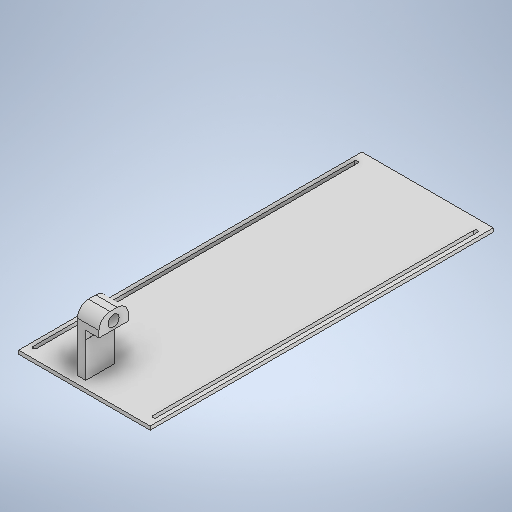
# Autodesk Inventor part: Part1
Saved by Autodesk Inventor 2025.2 (Build 292293000, 293)
## iProperties
Created: 2026-09-08
Part Number: Part1
Material: Generic
Document SubType Name: Sheet Metal
Designer: dguar
Density: 1 g/cm^3
Sheet Metal Rule: Default_mm
Appearance: Default
Author: dguar
Autodesk Inventor part; units mm, degrees
ref_plane "YZ Plane" through (0, 0, 0) normal (1, 0, 0) x (0, 1, 0)
ref_plane "XZ Plane" through (0, 0, 0) normal (0, 1, 0) x (-1, 0, 0)
ref_plane "XY Plane" through (0, 0, 0) normal (0, 0, 1) x (1, 0, 0)
sketch "Sketch1" plane through (0, 0, 0) normal (0, 1, 0) x (-1, 0, 0)
  line L0 (80, 0) -> (80, -250)
  line L1 (80, -250) -> (-80, -250)
  line L2 (-80, -250) -> (-80, 250)
  line L3 (-80, 250) -> (80, 250)
  line L4 (80, 250) -> (80, 0)
  point P0 (0, 0)
  constraints: 10 end point, 2 perpendicular, 1 point on line, 1 vertical
extrude "Extrusion1" add sketch "Sketch1" along normal blind 5
sketch "Sketch2" plane through (0, 5, 0) normal (0, 1, 0) x (1, 0, 0)
  line L0 (0, 0) -> (0, -200)
  line L1 (0, -200) -> (10, -200)
  line L2 (10, -200) -> (-10, -200)
  line L3 (-10, -200) -> (-10, -240)
  line L4 (-10, -240) -> (10, -240)
  line L5 (10, -240) -> (10, -200)
  dimension "d7" = 200
  dimension "d8" = 10
  dimension "d9" = 20
  dimension "d10" = 40
  dimension "d11" = 20
  constraints: 12 end point, 2 perpendicular, 1 horizontal, 1 point on line, 1 vertical
  measures "d7" distance of L0.start L0.end
  measures "d8" distance of L0.end L1.end
  measures "d9" distance of L1.end L2.end
  measures "d10" distance of L2.end L3.end
  measures "d11" distance of L3.end L4.end
extrude "Extrusion2" add sketch "Sketch2" along normal blind 100
sketch "Sketch3" plane through (10, 5, 240) normal (1, 0, 0) x (0, 0, -1)
  line L0 (40, 100) -> (0, 100) projected
  circle A0 centre (20, 70) radius 7.5
  point P0 (240, -5)
  dimension "d15" = 15
  constraints: 1 centre point
  measures "d15" diameter of A0
extrude "Extrusion3" cut sketch "Sketch3" against normal blind 100
sketch "Sketch4" plane through (80, 0, 250) normal (1, 0, 0) x (0, 0, -1)
  line L0 (0, 0) -> (0, 5) projected
  line L1 (0, 0) -> (500, 0) projected
  line L2 (0, 5) -> (500, 5)
  line L3 (500, 5) -> (500, 0)
  line L4 (500, 0) -> (0, 0)
  line L5 (0, 0) -> (0, 5)
  point P0 (250, 0)
  constraints: 8 end point, 2 parallel, 1 horizontal, 1 perpendicular
extrude "Extrusion4" add sketch "Sketch4" along normal blind 10
sketch "Sketch5" plane through (-80, 0, -250) normal (-1, 0, 0) x (0, 0, 1)
  line L0 (0, 5) -> (500, 5) projected
  line L1 (500, 0) -> (500, 5) projected
  line L2 (0, 5) -> (500, 5)
  line L3 (500, 5) -> (500, 0)
  line L4 (500, 0) -> (0, 0)
  line L5 (0, 0) -> (0, 5)
  point P0 (250, 0)
  constraints: 8 end point, 2 parallel, 1 horizontal, 1 perpendicular
extrude "Extrusion5" add sketch "Sketch5" along normal blind 10
sketch "Sketch6" plane through (90, 0, -250) normal (0, 0, -1) x (-1, 0, 0)
  line L0 (0, 5) -> (180, 5) projected
  line L1 (180, 0) -> (0, 0) projected
  line L2 (0, 5) -> (180, 5)
  line L3 (180, 5) -> (180, 0)
  line L4 (180, 0) -> (0, 0)
  line L5 (0, 0) -> (0, 5)
  point P0 (90, 0)
  constraints: 8 end point, 2 parallel, 1 horizontal, 1 perpendicular
extrude "Extrusion6" cut sketch "Sketch6" against normal blind 30
sketch "Sketch7" plane through (0, 5, 0) normal (0, 1, 0) x (1, 0, 0)
  line L0 (-90, -250) -> (90, -250) projected
  arc A0 (79.52, -235.7841) -> (84.52, -235.7841) centre (82.02, -235.7841) ccw
  arc A1 (84.52, 203.719) -> (79.52, 203.719) centre (82.02, 203.719) ccw
  line L1 (79.52, 203.719) -> (79.52, -235.7841)
  line L2 (84.52, -235.7841) -> (84.52, 203.719)
  line L3 (-90, -250) -> (-90, 220) projected
  line L4 (90, 220) -> (-90, 220) projected
  arc A2 (-79.52, 203.719) -> (-84.52, 203.719) centre (-82.02, 203.719) ccw
  arc A3 (-84.52, -235.7841) -> (-79.52, -235.7841) centre (-82.02, -235.7841) ccw
  line L5 (-84.52, -235.7841) -> (-84.52, 203.719)
  line L6 (-79.52, 203.719) -> (-79.52, -235.7841)
  point P0 (0, 0)
  dimension "d25" = 5
  dimension "d26" = 5
  dimension "d28" = 5
  dimension "d29" = 5
  constraints: 8 end point, 8 point on circle, 4 centre point, 4 tangent
  measures "d25" diameter of A0
  measures "d26" diameter of A1
  measures "d28" diameter of A2
  measures "d29" diameter of A3
extrude "Extrusion7" cut sketch "Sketch7" against normal blind 30
sketch "Sketch8" plane through (10, 5, 240) normal (1, 0, 0) x (0, 0, -1)
  point P0 (240, -5)
sketch "Sketch9" plane through (0, 105, 0) normal (0, 1, 0) x (1, 0, 0)
  line L0 (10, -240) -> (-10, -240) projected
  line L1 (-10, -200) -> (10, -200) projected
  line L2 (-10, -240) -> (10, -240)
  line L3 (10, -240) -> (10, -200)
  line L4 (10, -200) -> (-10, -200)
  line L5 (-10, -200) -> (-10, -240)
  point P0 (0, 0)
  constraints: 8 end point, 2 parallel, 1 horizontal, 1 perpendicular
extrude "Extrusion8" cut sketch "Sketch9" against normal blind 16.75
sketch "Sketch10" plane through (-10, 5, 200) normal (-1, 0, 0) x (0, 0, 1)
  line L0 (0, 0) -> (0, 83.25) projected
  line L1 (40, 0) -> (40, 83.25) projected
  line L2 (0, 83.25) -> (40, 83.25)
  line L3 (40, 83.25) -> (40, 0)
  line L4 (40, 0) -> (0, 0)
  line L5 (0, 0) -> (0, 83.25)
  circle A0 centre (20, 70) radius 7.5 projected
  circle A1 centre (20, 70) radius 7.5
  point P0 (-200, -5)
  constraints: 8 end point, 2 parallel, 1 centre point, 1 coincident, 1 horizontal, 1 perpendicular
extrude "Extrusion9" add sketch "Sketch10" along normal blind 9.5
sketch "Sketch11" plane through (10, 5, 200) normal (0, 0, -1) x (-1, 0, 0)
  line L0 (0, 0) -> (0, 83.25) projected
  line L1 (0, 0) -> (18.187, 0)
  line L2 (18.187, 0) -> (18.187, 48.2097)
  line L3 (18.187, 48.2097) -> (0, 48.2097)
  line L4 (0, 48.2097) -> (0, 0)
  point P0 (10, -5)
  constraints: 8 end point, 2 parallel, 1 horizontal, 1 perpendicular
extrude "Extrusion10" cut sketch "Sketch11" against normal blind 66.75
sketch "Sketch12" plane through (10, 88.25, 240) normal (1, 0, 0) x (0, 0, -1)
  line L0 (0, -83.25) -> (0, 0) projected
  line L1 (40, 0) -> (40, -83.25) projected
  line L2 (0, -35.059) -> (40, -35.059)
  line L3 (40, -35.059) -> (40, -23.8514)
  line L4 (40, -23.8514) -> (0, -23.8514)
  line L5 (0, -23.8514) -> (0, -35.059)
  point P0 (240, -88.25)
  constraints: 8 end point, 2 parallel, 2 point on line, 1 horizontal, 1 perpendicular
extrude "Extrusion11" cut sketch "Sketch12" against normal blind 18.25
fillet "Fillet1" radius 15 2 edges at (-4.75, 88.25, 240) (-4.75, 88.25, 200)
equation "\"BendRadius\" = Thickness"
equation "\"BendReliefWidth\" = Thickness"
equation "\"BendReliefDepth\" = 0.5 * Thickness"
equation "\"CornerReliefSize\" = 4 * Thickness"
equation "\"MinimumRemnant\" = 2 * Thickness"
equation "\"TransitionRadius\" = BendRadius"
equation "\"JacobiRadiusSize\" = BendRadius"
equation "\"GapSize\" = Thickness"
equation "\"Thickness\" = 0.5"
body "Solid1"
